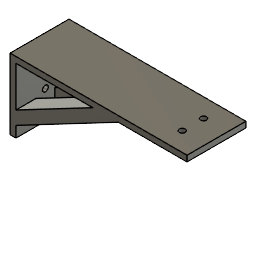
Base Bracket (Autodesk Fusion 360 design; units mm, degrees)
Autodesk Fusion 360 part; units mm, degrees
sketch "Sketch1" plane through (0, 0, 0) normal (0, 0, 1) x (1, 0, 0)
  line L0 (0, 0) -> (5, 0)
  line L1 (0, 60) -> (0, 0)
  line L2 (0, 60) -> (150, 60)
  line L3 (150, 60) -> (150, 55)
  line L4 (5, 9.3963) -> (91.6413, 55)
  line L5 (5, 9.3963) -> (91.6413, 55)
  line L6 (70.1715, 55) -> (5, 20.6969)
  line L7 (5, 0) -> (5, 9.3963)
  line L8 (5, 20.6969) -> (5, 55)
  line L9 (150, 55) -> (91.6413, 55)
  line L10 (70.1715, 55) -> (5, 55)
  dimension "d1" = 5
  dimension "d2" = 60
  dimension "d3" = 150
  dimension "d9" = 5
  dimension "d10" = 10
  constraint horizontal L0
  constraint vertical L7
  constraint vertical L1
  constraint coincident L0.start L1.end
  constraint horizontal L2
  constraint vertical L3
  constraint horizontal L9
  constraint parallel L5 L6
  constraint coincident L6.start L9
  constraint coincident L6.end L7
  constraint collinear L7 L8
  constraint collinear L9 L10
  measures "d1" distance of L0.start L0.end
  measures "d2" distance of L0.start L1.start
  measures "d3" distance of L1.start L2.end
  measures "d9" distance of L2 L9
  measures "d10" distance of L5 L6
extrude "Extrude1" add sketch "Sketch1" along normal blind 50
sketch "Sketch2" plane through (-2.7881, 5.297, 0) normal (0.465771, -0.884905, 0) x (0, 0, -1)
  line L0 (0, 8.801) -> (0, 106.7113)
  line L1 (0, 106.7113) -> (-50, 106.7113)
  line L2 (-50, 106.7113) -> (-50, 8.801)
  line L3 (-50, 8.801) -> (0, 8.801)
  line L4 (-33, 106.7113) -> (-17, 106.7113)
  line L5 (-17, 106.7113) -> (-17, 8.801)
  line L6 (-17, 8.801) -> (-33, 8.801)
  line L7 (-33, 8.801) -> (-33, 106.7113)
  dimension "d11" = 16
  constraint vertical L5
  constraint vertical L7
  constraint collinear L3 L6
  constraint collinear L1 L4
  constraint midpoint L1 L4
  measures "d11" distance of L5 L7
sketch "Sketch3" plane through (-7.4458, 14.1461, 0) normal (-0.465771, 0.884905, 0) x (0, 0, 1)
  line L0 (0, 87.7125) -> (0, 14.0645)
  line L1 (0, 14.0645) -> (50, 14.0645)
  line L2 (50, 14.0645) -> (50, 87.7125)
  line L3 (50, 87.7125) -> (0, 87.7125)
  line L4 (33, 8.801) -> (33, 106.7113)
  line L5 (17, 106.7113) -> (17, 8.801)
extrude "Extrude2" cut sketch "Sketch3" against normal blind 10 contours L1 L3 L4 L5
sketch "Sketch5" plane through (0, 0, 0) normal (0, 1, 0) x (1, 0, 0)
  line L0 (5, -17) -> (91.6413, -17)
  line L1 (91.6413, -17) -> (91.6413, -33)
  line L2 (91.6413, -33) -> (5, -33)
  line L3 (5, -33) -> (5, -17)
  line L4 (5, 0) -> (5, -50)
  line L5 (91.6413, 0) -> (91.6413, -50)
  dimension "d17" = 16
  dimension "d18" = 5
  constraint horizontal L0
  constraint vertical L1
  constraint horizontal L2
  constraint vertical L3
  constraint collinear L1 L5
  measures "d17" distance of L0.start L2.end
  measures "d18" distance of origin L3
extrude "Extrude3" cut sketch "Sketch5" along normal blind 55
sketch "Sketch4" plane through (5, 0, 0) normal (1, 0, 0) x (0, 0, -1)
  line L0 (0, 0) -> (0, 9.3963)
  line L1 (0, 55) -> (-50, 55)
  line L2 (-50, 55) -> (-50, 20.6969)
  line L3 (-50, 20.6969) -> (-33, 20.6969)
  line L4 (-17, 20.6969) -> (0, 20.6969)
  circle A0 centre (-25, 8) radius 2.5
  circle A1 centre (-25, 24) radius 2.5
  line L5 (-50, 0) -> (0, 0)
  line L6 (0, 9.3963) -> (-17, 9.3963)
  line L7 (-17, 9.3963) -> (-17, 20.6969)
  line L8 (-33, 20.6969) -> (-33, 9.3963)
  line L9 (-33, 9.3963) -> (-50, 9.3963)
  line L10 (-50, 9.3963) -> (-50, 0)
  line L11 (0, 20.6969) -> (0, 55)
  dimension "d14" = 5
  dimension "d22" = 5
  dimension "d23" = 16
  measures "d14" diameter of A0
  measures "d22" diameter of A1
  measures "d23" distance of A0.centre A1.centre
extrude "Extrude4" cut sketch "Sketch4" against normal blind 10 contours A0 | A1
sketch "Sketch6" plane through (0, 55, 0) normal (0, -1, 0) x (1, 0, 0)
  line L0 (91.6413, 0) -> (150, 0)
  line L1 (150, 0) -> (150, 50)
  line L2 (150, 50) -> (91.6413, 50)
  line L3 (91.6413, 50) -> (91.6413, 33)
  circle A0 centre (130, 34) radius 2.5
  circle A1 centre (130, 16) radius 2.5
  line L4 (91.6413, 33) -> (70.1715, 33)
  line L5 (70.1715, 33) -> (70.1715, 50)
  line L6 (70.1715, 50) -> (5, 50)
  line L7 (5, 50) -> (5, 0)
  line L8 (5, 0) -> (70.1715, 0)
  line L9 (70.1715, 0) -> (70.1715, 17)
  line L10 (70.1715, 17) -> (91.6413, 17)
  line L11 (91.6413, 17) -> (91.6413, 0)
  dimension "d26" = 5
  dimension "d27" = 20
  dimension "d29" = 5
  dimension "d32" = 16
  dimension "d33" = 16
  measures "d26" diameter of A0
  measures "d27" distance of L1 A0.centre
  measures "d29" diameter of A1
  measures "d32" distance of L2 A0.centre
  measures "d33" distance of L0 A1.centre
extrude "Extrude5" cut sketch "Sketch6" against normal blind 10 contours A0 | A1
